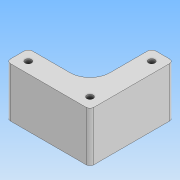
# Autodesk Inventor part: stepper spacer
Saved by Autodesk Inventor 2020 (Build 240168000, 168)
## iProperties
Created: 2020-05-18
Part Number: stepper spacer
Material: Generic
Document SubType Name: Modeling
Designer: stefa
Density: 1 g/cm^3
Appearance: Default
Author: stefa
Autodesk Inventor part; units mm, degrees
ref_plane "YZ Plane" through (0, 0, 0) normal (1, 0, 0) x (0, 1, 0)
ref_plane "XZ Plane" through (0, 0, 0) normal (0, 1, 0) x (-1, 0, 0)
ref_plane "XY Plane" through (0, 0, 0) normal (0, 0, 1) x (1, 0, 0)
sketch "Sketch1" plane through (0, 0, 0) normal (0, 1, 0) x (-1, 0, 0)
  line L0 (0, 19) -> (0, -19)
  line L1 (21, 10) -> (40, 10)
  line L2 (42, 12) -> (42, 19)
  line L3 (40, 21) -> (2, 21)
  arc A0 (42, 19) -> (40, 21) centre (40, 19) ccw
  arc A1 (40, 10) -> (42, 12) centre (40, 12) ccw
  arc A2 (2, 21) -> (0, 19) centre (2, 19) ccw
  circle A3 centre (5.5, 15.5) radius 1.6
  circle A4 centre (36.5, 15.5) radius 1.6
  circle A5 centre (5.5, -15.5) radius 1.6
  line L4 (9, -21) -> (2, -21)
  arc A6 (0, -19) -> (2, -21) centre (2, -19) ccw
  line L5 (11, -19) -> (11, 0)
  arc A7 (9, -21) -> (11, -19) centre (9, -19) ccw
  arc A8 (21, 10) -> (11, 0) centre (21, 0) ccw
  point P0 (0, 21)
  point P1 (0, -8.7206)
  point P2 (42, 10)
  point P3 (42, 21)
  point P4 (0, -21)
  point P5 (42, 15.5)
  point P6 (0, 0)
  point P7 (0, 0)
  dimension "d4" = 11
  dimension "d7" = 2
  dimension "d8" = 3.2
  dimension "d21" = 5.5
  dimension "d22" = 31
  dimension "d23" = 31
  dimension "d29" = 2
  dimension "d30" = 42
  dimension "d32" = 2
  dimension "d33" = 10
  constraints: 12 end point, 12 point on circle, 12 tangent, 9 centre point, 9 point on line, 4 equal radius, 3 perpendicular, 2 coincident, 2 horizontal alignment, 2 midpoint, 2 parallel, 2 vertical, 1 horizontal, 1 vertical alignment
  measures "d4" distance of point (42, 10) point (42, 21)
  measures "d7" radius of A0
  measures "d8" diameter of A3
  measures "d21" distance from line of L0 A3.centre
  measures "d22" distance of A5.centre A3.centre
  measures "d23" distance of A4.centre A3.centre
  measures "d29" radius of A6
  measures "d30" distance between parallel lines of L4 L3
  measures "d32" radius of A7
  measures "d33" radius of A8
extrude "Extrusion1" add sketch "Sketch1" along normal blind 25
body "Solid1"
